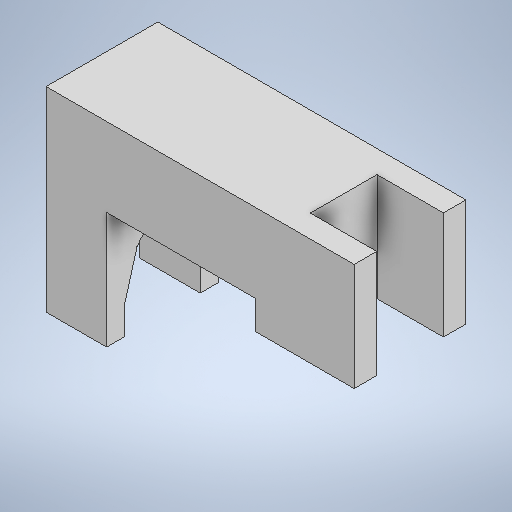
# Autodesk Inventor part: Holder2
Saved by Autodesk Inventor 2025.1 (Build 291241000, 241)
## iProperties
Created: 2024-10-19
Part Number: Holder2
Material: Generic
Document SubType Name: Modeling
Designer: 13156
Density: 1 g/cm^3
Appearance: Default
Author: 13156
Autodesk Inventor part; units mm, degrees
ref_plane "YZ Plane" through (0, 0, 0) normal (1, 0, 0) x (0, 1, 0)
ref_plane "XZ Plane" through (0, 0, 0) normal (0, 1, 0) x (-1, 0, 0)
ref_plane "XY Plane" through (0, 0, 0) normal (0, 0, 1) x (1, 0, 0)
sketch "Sketch1" plane through (0, 0, 0) normal (1, 0, 0) x (0, 1, 0)
  line L0 (-5.8, 12.5) -> (-15, 12.5)
  line L1 (-5.8, -12.5) -> (-15, -12.5)
  line L2 (-5.8, 12.5) -> (8.7, 8.35)
  line L3 (-5.8, -12.5) -> (8.7, -8.35)
  arc A0 (8.7, -8.35) -> (8.7, 8.35) centre (3.8372, 0) ccw
  line L4 (-15, 12.5) -> (-15, 18.5)
  line L5 (-15, 18.5) -> (23.5, 18.5)
  line L6 (23.5, 18.5) -> (23.5, -18.5)
  line L7 (23.5, -18.5) -> (-15, -18.5)
  line L8 (-15, -18.5) -> (-15, -12.5)
  point P0 (0, 0)
  point P1 (-10.4, 12.5)
  point P2 (10.8853, -1.4818)
  point P3 (13.5, 0)
  point P4 (23.5, 0)
  dimension "d0" = 9.2
  dimension "d1" = 25
  dimension "d2" = 12.5
  dimension "d5" = 14.5
  dimension "d6" = 14.5
  dimension "d7" = 9.2
  dimension "d8" = 12.5
  dimension "d9" = 15
  dimension "d10" = 15
  dimension "d11" = 4.15
  dimension "d12" = 4.15
  dimension "d13" = 4.8
  dimension "d14" = 6
  dimension "d15" = 6
  dimension "d16" = 37
  dimension "d29" = 10
  constraints: 18 end point, 3 perpendicular, 3 point on circle, 2 horizontal, 2 midpoint, 1 centre point, 1 point on line, 1 vertical
  measures "d0" distance of L0.start L0.end
  measures "d1" distance between parallel lines of L1 L0
  measures "d2" vertical distance of point (-10.4, 12.5) point (0, 0)
  measures "d5" horizontal distance of L0.start L2.end
  measures "d6" horizontal distance of L1.start L3.end
  measures "d7" distance of L1.start L1.end
  measures "d8" vertical distance of L1.start point (0, 0)
  measures "d9" horizontal distance of L1.end point (0, 0)
  measures "d10" horizontal distance of point (0, 0) L0.end
  measures "d11" vertical distance of L1.start L3.end
  measures "d12" vertical distance of L2.end L0.start
  measures "d13" horizontal distance of L3.end point (13.5, 0)
  measures "d14" distance of L0.end L4.end
  measures "d15" distance of L7.end L1.end
  measures "d16" distance of L5.end L6.end
  measures "d29" distance of point (23.5, 0) point (13.5, 0)
extrude "Extrusion1" add sketch "Sketch1" along normal blind 20
sketch "Sketch2" plane through (0, 23.5, 18.5) normal (0, 1, 0) x (1, 0, 0)
  line L0 (0, 31) -> (0, 37) projected
  line L1 (0, 37) -> (80, 37)
  line L2 (80, 37) -> (80, 0.0995)
  line L3 (80, 0.0995) -> (0, 0.0995)
  line L4 (0, 0.0995) -> (0, 37)
  line L5 (20, 37) -> (20, 0) projected
  point P0 (0, 18.5)
  point P1 (80, 18.5498)
  point P2 (0, 31)
  dimension "d19" = 60
  constraints: 8 end point, 2 parallel, 1 horizontal, 1 midpoint, 1 perpendicular
  measures "d19" distance from line of L5 point (80, 18.55)
extrude "Extrusion2" add sketch "Sketch2" along normal blind 10
sketch "Sketch3" plane through (0, 23.5, 18.5) normal (0, -1, 0) x (1, 0, 0)
  line L0 (120.5, -8.5498) -> (120.5, -28.5498)
  line L1 (120.5, -28.5498) -> (80, -28.5498)
  line L2 (80, -28.5498) -> (80, -8.5498)
  line L3 (80, -0.0995) -> (80, -37) projected
  line L4 (120.5, -8.5498) -> (129.5, -8.5498)
  line L5 (129.5, -8.5498) -> (129.5, -37)
  line L6 (129.5, -37) -> (80, -37)
  line L7 (80, -37) -> (0, -37) projected
  line L8 (80, -37) -> (69, -37)
  line L9 (69, -37) -> (69, -8.5498)
  line L10 (69, -8.5498) -> (80, -8.5498)
  point P0 (0, -18.5)
  point P1 (80, -18.5498)
  point P2 (80, -18.5498)
  point P3 (120.5, -18.5498)
  dimension "d22" = 20
  dimension "d23" = 20
  dimension "d24" = 0
  dimension "d25" = 40.5
  dimension "d26" = 9
  dimension "d30" = 11
  constraints: 18 end point, 4 perpendicular, 3 midpoint, 2 point on line, 2 vertical, 1 horizontal
  measures "d22" distance of L0.start L0.end
  measures "d23" distance of L1.end L2.end
  measures "d24" distance of point (80, -18.55) point (80, -18.55)
  measures "d25" distance from line of L2 point (120.5, -18.55)
  measures "d26" distance between parallel lines of L0 L5
  measures "d30" distance between parallel lines of L9 L2
extrude "Extrusion3" add sketch "Sketch3" along normal blind 9.5 and the other way blind 10
sketch "Sketch4" plane through (0, 33.5, 18.5) normal (0, 1, 0) x (1, 0, 0)
  line L0 (120.5, 8.5498) -> (129.5, 8.5498) projected
  line L1 (72.5, 28.5653) -> (129.5, 28.5653)
  line L2 (129.5, 28.5653) -> (129.5, 8.5498)
  line L3 (129.5, 8.5498) -> (72.5, 8.5498)
  line L4 (72.5, 8.5498) -> (72.5, 28.5653)
  line L5 (80, 0.0995) -> (80, 28.5498) projected
  line L6 (120.5, 28.5498) -> (120.5, 8.5498) projected
  point P0 (0, 18.5)
  point P1 (80, 14.3246)
  dimension "d33" = 7.5
  dimension "d34" = 9
  constraints: 8 end point, 2 parallel, 1 horizontal, 1 midpoint, 1 perpendicular, 1 point on line
  measures "d33" distance from line of point (80, 14.325) L4
  measures "d34" distance between parallel lines of L6 L2
extrude "Extrusion4" cut sketch "Sketch4" against normal blind 14.2625
sketch "Sketch5" plane through (0, 33.5, 18.5) normal (0, 1, 0) x (1, 0, 0)
  line L0 (72.5, 8.5498) -> (72.5, 28.5653) projected
  line L1 (72.5, 8.5498) -> (80, 8.5498)
  line L2 (80, 8.5498) -> (80, -1.0168)
  line L3 (80, -1.0168) -> (72.5, -1.0168)
  line L4 (72.5, -1.0168) -> (72.5, 8.5498)
  line L5 (80, 0.0995) -> (80, 8.5498) projected
  point P0 (0, 18.5)
  dimension "d47" = 0
  constraints: 8 end point, 2 parallel, 1 horizontal, 1 perpendicular
  measures "d47" distance between parallel lines of L2 L5
extrude "Extrusion5" cut sketch "Sketch5" against normal blind 14.2625
sketch "Sketch7" plane through (69, 14, 9.9502) normal (0, 0, 1) x (1, 0, 0)
  line L0 (3.5, 5.2375) -> (3.5, 9.5) projected
  line L1 (11, 0) -> (11, 5.2375) projected
  line L2 (3.5, 5.2375) -> (11, 5.2375)
  line L3 (11, 5.2375) -> (11, 0)
  line L4 (11, 0) -> (0, 0)
  line L5 (0, 0) -> (0, 9.5)
  line L6 (0, 9.5) -> (3.5, 9.5)
  line L7 (-49, 9.5) -> (3.5, 9.5) projected
  line L8 (3.5, 9.5) -> (3.5, 19.5) projected
  point P0 (-69, -14)
  dimension "d42" = 11
  dimension "d43" = 0
  dimension "d44" = 0
  constraints: 10 end point, 3 perpendicular, 1 collinear, 1 horizontal
  measures "d42" distance of L1.start L4.end
  measures "d43" distance between parallel lines of L7 L6
  measures "d44" distance from line of L8 L6.end
extrude "Extrusion7" add sketch "Sketch7" along normal blind 8.45
sketch "Sketch8" plane through (72.5, 33.5, 18.4005) normal (1, 0, 0) x (0, 0, -1)
  line L0 (28.4658, 0) -> (28.4658, -14.2625) projected
  line L1 (36.9005, 0) -> (0, 0) projected
  line L2 (28.4658, -9.8625) -> (0, -9.8625)
  line L3 (0, -9.8625) -> (0, 0)
  line L4 (0, 0) -> (28.4658, 0)
  line L5 (28.4658, 0) -> (28.4658, -9.8625)
  line L6 (28.4658, -14.2625) -> (8.4502, -14.2625) projected
  line L7 (8.4502, -14.2625) -> (8.4502, -19.5) projected
  line L8 (0, -10) -> (0, 0) projected
  point P0 (18.4005, -33.5)
  dimension "d48" = 4.4
  dimension "d52" = 0
  constraints: 8 end point, 2 parallel, 2 point on line, 1 horizontal, 1 perpendicular
  measures "d48" distance between parallel lines of L2 L6
  measures "d52" distance between parallel lines of L8 L3
extrude "Extrusion8" add sketch "Sketch8" along normal blind 7.5
sketch "Sketch9" plane through (0, 33.5, 18.5) normal (0, 1, 0) x (1, 0, 0)
  line L0 (69, 37) -> (69, 0.0998) projected
  line L1 (69, 0.0998) -> (69, 37)
  line L2 (129.5, 37) -> (129.5, 8.5498) projected
  line L3 (69, 37) -> (129.5, 37)
  line L4 (80, 28.5653) -> (129.5, 28.5653) projected
  line L5 (129.5, 37) -> (129.5, 28.5653)
  line L6 (129.5, 28.5653) -> (80, 28.5653)
  line L7 (0, 0.0995) -> (80, 0.0995) projected
  line L8 (80, 28.5653) -> (80, 0.0995)
  line L9 (80, 0.0995) -> (69, 0.0998)
  point P0 (0, 18.5)
  constraints: 12 end point, 3 perpendicular, 2 collinear
extrude "Extrusion9" add sketch "Sketch9" along normal blind 16
sketch "Sketch10" plane through (0, 33.5, 18.5) normal (0, 1, 0) x (1, 0, 0)
  line L0 (69, 0.0998) -> (69, 37) projected
  line L1 (0, 0.0995) -> (80, 0.0995) projected
  line L2 (69, 37) -> (0, 37)
  line L3 (0, 37) -> (0, 0.0995)
  line L4 (0, 0.0995) -> (69, 0.0995)
  line L5 (69, 0.0995) -> (69, 37)
  point P0 (0, 18.5)
  point P1 (69, 0.0995)
  constraints: 8 end point, 2 parallel, 1 horizontal, 1 perpendicular
extrude "Extrusion10" add sketch "Sketch10" along normal blind 16
sketch "Sketch12" plane through (0, 49.5, 18.5) normal (0, 1, 0) x (1, 0, 0)
  line L0 (80, 28.5498) -> (80, 0.0998) projected
  line L1 (80, 0.0998) -> (-1.6844, 0.0998)
  line L2 (-1.6844, 0.0998) -> (-1.6844, -16.6848)
  line L3 (-1.6844, -16.6848) -> (80, -16.6848)
  line L4 (80, -16.6848) -> (80, 0.0998)
  point P0 (0, 18.5)
  constraints: 8 end point, 2 parallel, 1 horizontal, 1 perpendicular
extrude "Extrusion11" cut sketch "Sketch12" against normal blind 76.325
sketch "Sketch13" plane through (0, 19.2375, 18.5) normal (0, 1, 0) x (1, 0, 0)
  line L0 (120.5, 8.5498) -> (120.5, 28.5498) projected
  line L1 (80, 0.0998) -> (80, 28.5653) projected
  line L2 (120.5, 28.5498) -> (80, 28.5498)
  line L3 (80, 28.5498) -> (80, 28.5653)
  line L4 (80, 28.5653) -> (120.5, 28.5653)
  line L5 (120.5, 28.5653) -> (120.5, 28.5498)
  point P0 (0, 18.5)
  constraints: 8 end point, 2 parallel, 1 horizontal, 1 perpendicular
extrude "Extrusion12" cut sketch "Sketch13" against normal blind 76.325
sketch "Sketch14" plane through (0, 14, 18.5) normal (0, -1, 0) x (1, 0, 0)
  circle A0 centre (124.7, -23.3) radius 2.1
  circle A1 centre (124.7, -13.2) radius 2.1
  line L0 (120.5, -8.5498) -> (120.5, -28.5653) projected
  line L1 (20, -10.15) -> (20, -26.85) projected
  point P0 (0, -18.5)
  point P1 (20, -18.5)
  dimension "d61" = 4.2
  dimension "d62" = 4.2
  dimension "d63" = 10.1
  dimension "d64" = 4.2
  dimension "d65" = 0
  dimension "d66" = 4.8
  constraints: 2 centre point, 1 midpoint
  measures "d61" diameter of A0
  measures "d62" diameter of A1
  measures "d63" distance of A0.centre A1.centre
  measures "d64" distance from line of L0 A0.centre
  measures "d65" horizontal distance of A0.centre A1.centre
  measures "d66" vertical distance of point (20, -18.5) A0.centre
extrude "Extrusion13" cut sketch "Sketch14" against normal blind 12.825
pattern_linear "Rectangular Pattern1" count 2 spacing 49 along (-1, 0, 0) of "Extrusion13"
sketch "Sketch15" plane through (0, 14, 18.5) normal (0, -1, 0) x (1, 0, 0)
  line L0 (80, -0.0998) -> (80, -28.5653) projected
  line L1 (80, -0.0998) -> (129.5, -0.0998)
  line L2 (129.5, -0.0998) -> (129.5, -8.5498)
  line L3 (129.5, -8.5498) -> (120.5, -8.5498) projected
  line L4 (129.5, -8.5498) -> (120.5, -8.5498)
  line L5 (120.5, -8.5498) -> (78.2571, -8.5498)
  line L6 (78.2571, -8.5498) -> (69, -8.5498)
  line L7 (69, -37) -> (69, -0.0998) projected
  line L8 (69, -0.0998) -> (69, -8.5498)
  line L9 (69, -0.0998) -> (80, -0.0998)
  point P0 (0, -18.5)
  constraints: 14 end point, 4 point on line, 3 perpendicular, 1 collinear, 1 horizontal
extrude "Extrusion14" add sketch "Sketch15" against normal blind 35.5
sketch "Sketch16" plane through (129.5, 14, 18.4002) normal (1, 0, 0) x (0, 0, -1)
  line L0 (7.45, 5.2375) -> (29.4655, 5.2375)
  line L1 (29.4655, 5.2375) -> (29.4655, 38.0522)
  line L2 (29.4655, 38.0522) -> (7.45, 38.0522)
  line L3 (7.45, 38.0522) -> (7.45, 5.2375)
  line L4 (28.4655, 5.2375) -> (8.45, 5.2375) projected
  line L5 (8.45, 5.2375) -> (8.45, 35.5) projected
  line L6 (28.4655, 35.5) -> (28.4655, 5.2375) projected
  point P0 (18.4002, -14)
  dimension "d74" = 0
  dimension "d75" = 1
  dimension "d76" = 1
  constraints: 8 end point, 2 parallel, 1 horizontal, 1 perpendicular
  measures "d74" distance between parallel lines of L4 L0
  measures "d75" distance between parallel lines of L5 L3
  measures "d76" distance between parallel lines of L6 L1
extrude "Extrusion15" cut sketch "Sketch16" against normal blind 49.6875
sketch "Sketch19" plane through (0, 14, 18.5) normal (0, -1, 0) x (1, 0, 0)
  line L0 (134.9623, 3.6486) -> (101.7268, 3.6486)
  line L1 (101.7268, 3.6486) -> (101.7268, -43.9762)
  line L2 (101.7268, -43.9762) -> (134.9623, -43.9762)
  line L3 (134.9623, -43.9762) -> (134.9623, 3.6486)
  point P0 (0, -18.5)
  constraints: 8 end point, 2 parallel, 1 horizontal, 1 perpendicular
extrude "Extrusion18" cut sketch "Sketch19" against normal blind 65.5625
sketch "Sketch20" plane through (0, 49.5, 18.5) normal (0, 1, 0) x (1, 0, 0)
  line L0 (101.7268, 28.5653) -> (101.7268, 29.5653) projected
  line L1 (101.7268, 7.5498) -> (79.8125, 7.5498) projected
  line L2 (101.7268, 29.5653) -> (79.8125, 29.5653)
  line L3 (79.8125, 29.5653) -> (79.8125, 7.5498)
  line L4 (79.8125, 7.5498) -> (101.7268, 7.5498)
  line L5 (101.7268, 7.5498) -> (101.7268, 29.5653)
  point P0 (0, 18.5)
  constraints: 8 end point, 2 parallel, 1 horizontal, 1 perpendicular
extrude "Extrusion19" cut sketch "Sketch20" against normal blind 65.5625
body "Solid1"
